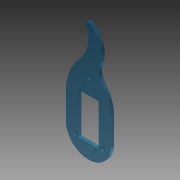
# Autodesk Inventor part: tail_top
Saved by Autodesk Inventor 2015 SP2 (Build 190223200, 223)
## iProperties
Created: 2015-10-08
Part Number: tail_top
Material: Generic
Document SubType Name: Modeling
Designer: styku
Density: 1 g/cm^3
Appearance: Clear
Author: styku
Autodesk Inventor part; units mm, degrees
ref_plane "YZ Plane" through (0, 0, 0) normal (1, 0, 0) x (0, 1, 0)
ref_plane "XZ Plane" through (0, 0, 0) normal (0, 1, 0) x (-1, 0, 0)
ref_plane "XY Plane" through (0, 0, 0) normal (0, 0, 1) x (1, 0, 0)
sketch "Sketch1" plane through (0, 0, 0) normal (0, 1, 0) x (-1, 0, 0)
  line L0 (46, 0) -> (-35, 0) construction
  line L1 (0, 54.3949) -> (0, -60) construction
  line L2 (10, 20) -> (-10, 20)
  line L3 (-10, 20) -> (-10, -20)
  line L4 (-10, -20) -> (10, -20)
  line L5 (10, -20) -> (10, 20)
  line L6 (22, -12.5) -> (22, 12.5)
  circle A0 centre (5, 24.25) radius 0.5
  circle A1 centre (-5, 24.25) radius 0.5
  line L7 (14.6784, 24.25) -> (-18, 24.25) construction
  circle A2 centre (5, -24.25) radius 0.5
  circle A3 centre (-5, -24.25) radius 0.5
  circle A4 centre (13.5, -18.75) radius 1.5
  line L8 (-22, 12.5) -> (-22, -12.5)
  circle A5 centre (0, 35) radius 1.5
  circle A6 centre (-13.5, -18.75) radius 1.5
  arc A7 (-22, -12.5) -> (22, -12.5) centre (0, -12) ccw
  arc A8 (-13.5294, 35.6977) -> (-11.0832, 50.96) centre (-25, 45.3634) ccw
  arc A9 (-13.5294, 35.6977) -> (-22, 12.5) centre (14, 12.5) ccw
  arc A10 (2.3262, 78.3342) -> (-1.3457, 81.3569) centre (0, 79.25) ccw
  arc A11 (-1.3457, 81.3569) -> (-11.0832, 50.96) centre (12.1114, 60.2879) ccw
  arc A12 (2.3262, 78.3342) -> (8.4007, 46.7782) centre (30.2411, 67.345) ccw
  arc A13 (22, 12.5) -> (8.4007, 46.7782) centre (-28, 12.5) ccw
  arc A14 (22, 12.5) -> (22, 12.5) centre (42.4714, 12.5) ccw
  point P0 (0, 0)
  dimension "d0" = 40
  dimension "d1" = 20
  dimension "d2" = 12
  dimension "d6" = 20
  dimension "d7" = 10
  dimension "d11" = 1
  dimension "d12" = 1
  dimension "d13" = 5
  dimension "d14" = 5
  dimension "d15" = 4.25
  dimension "d16" = 3
  dimension "d29" = 3.5
  dimension "d44" = 3
  dimension "d49" = 15
  dimension "d50" = 1.25
  dimension "d53" = 12
  dimension "d54" = 25
  dimension "d56" = 5
  dimension "d57" = 15
  dimension "d58" = 36
  dimension "d59" = 50
  dimension "d60" = 25
  dimension "d61" = 30
  dimension "d62" = 0
  dimension "d63" = 55
  dimension "d64" = 25
  constraints: 18 end point, 17 point on circle, 15 centre point, 9 tangent, 4 point on line, 4 symmetric about line, 4 vertical, 3 horizontal, 3 perpendicular, 1 parallel, 4 other
  measures "d0" distance between parallel lines of L4 L2
  measures "d1" distance between parallel lines of L3 L5
  measures "d2" distance between parallel lines of L5 L6
  measures "d6" distance between parallel lines of L0 L2
  measures "d7" distance between parallel lines of L1 L5
  measures "d11" diameter of A1
  measures "d12" diameter of A0
  measures "d13" distance from line of A0.centre L5
  measures "d14" distance from line of L3 A1.centre
  measures "d15" distance between parallel lines of L2 L7
  measures "d16" diameter of A4
  measures "d29" distance from line of L5 A4.centre
  measures "d44" diameter of A5
  measures "d49" distance from line of L2 A5.centre
  measures "d50" distance from line of L4 A6.centre
  measures "d53" distance from line of L0 A7.centre
  measures "d54" distance of L8.start L8.end
  measures "d56" diameter of A10
  measures "d57" radius of A8
  measures "d58" radius of A9
  measures "d59" radius of A13
  measures "d60" radius of A11
  measures "d61" radius of A12
  measures "d62" distance from line of L1 A10.centre
  measures "d63" distance from line of L7 A10.centre
  measures "d64" distance from line of L1 A8.centre
extrude "Extrusion3" add sketch "Sketch1" along normal blind 3 contours A7 L8 A9 A8 A11 A10 A12 A13 L6
body "Solid3"
